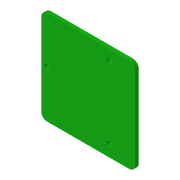
# Autodesk Inventor part: breadbord_2_inch
Saved by Autodesk Inventor 2018 (Build 220112000, 112)
## iProperties
Created: 2019-04-30
Part Number: breadbord_2_inch
Material: Generic
Document SubType Name: Modeling
Designer: amink
Density: 1 g/cm^3
Appearance: Default
Author: amink
Autodesk Inventor part; units mm, degrees
ref_plane "YZ Plane" through (0, 0, 0) normal (1, 0, 0) x (0, 1, 0)
ref_plane "XZ Plane" through (0, 0, 0) normal (0, 1, 0) x (-1, 0, 0)
ref_plane "XY Plane" through (0, 0, 0) normal (0, 0, 1) x (1, 0, 0)
sketch "Sketch1" plane through (0, 0, 0) normal (0, 0, 1) x (1, 0, 0)
  line L0 (-25.4, 25.4) -> (25.4, 25.4)
  line L1 (25.4, 25.4) -> (25.4, -25.4)
  line L2 (25.4, -25.4) -> (-25.4, -25.4)
  line L3 (-25.4, -25.4) -> (-25.4, 25.4)
  point P0 (0, 0)
  dimension "d0" = 25.4
  dimension "d1" = 50.8
  dimension "d2" = 50.8
  dimension "d3" = 25.4
  constraints: 8 end point, 2 parallel, 1 horizontal, 1 perpendicular
  measures "d0" distance from line of point (0, 0) L3
  measures "d1" distance between parallel lines of L1 L3
  measures "d2" distance between parallel lines of L2 L0
  measures "d3" distance from line of point (0, 0) L2
extrude "Extrusion1" add sketch "Sketch1" along normal blind 2
fillet "Fillet1" radius 3.175 4 edges at (25.4, 25.4, 1) (25.4, -25.4, 1) (-25.4, 25.4, 1) (-25.4, -25.4, 1)
sketch "Sketch2" plane through (0, 0, 2) normal (0, 0, 1) x (1, 0, 0)
  circle A0 centre (-22.4, -0.0994) radius 1.5
  circle A1 centre (11.4, -19.4) radius 1.5
  circle A2 centre (11.4, 19.4) radius 1.5
  line L0 (-25.4, 22.225) -> (-25.4, -22.225) projected
  line L1 (22.225, 25.4) -> (-22.225, 25.4) projected
  line L2 (-22.225, -25.4) -> (22.225, -25.4) projected
  line L3 (25.4, -22.225) -> (25.4, 22.225) projected
  point P0 (0, 0)
  dimension "d7" = 3
  dimension "d9" = 3
  dimension "d17" = 3
  dimension "d18" = 6
  dimension "d19" = 6
  dimension "d20" = 14
  dimension "d21" = 14
  dimension "d22" = 3
  constraints: 3 centre point
  measures "d7" diameter of A0
  measures "d9" diameter of A1
  measures "d17" distance from line of L0 A0.centre
  measures "d18" distance from line of L1 A2.centre
  measures "d19" distance from line of L2 A1.centre
  measures "d20" distance from line of L3 A2.centre
  measures "d21" distance from line of L3 A1.centre
  measures "d22" diameter of A2
extrude "Extrusion2" cut sketch "Sketch2" against normal blind 2
equation "\"d0\" = 0.5 * d1"
equation "\"d3\" = 0.5 * d2"
equation "\"d9\" = d7"
equation "\"d19\" = d18"
equation "\"d21\" = d20"
equation "\"d22\" = d7"
body "Solid1"
